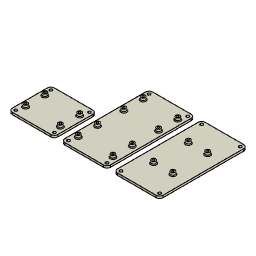
Lower Bay Tray - Parametric Mount Generator (Autodesk Fusion 360 design; units mm, degrees)
Autodesk Fusion 360 part; units mm, degrees
sketch "Base Sketch" plane through (0, 0, 0) normal (0, 0, 1) x (1, 0, 0)
  line L0 (-65, 70) -> (-10, 70) construction
  line L1 (-10, 70) -> (-10, 20) construction
  line L2 (-10, 20) -> (-65, 20) construction
  line L3 (-65, 20) -> (-65, 70) construction
  line L4 (-70, 20) -> (-70, 70)
  arc A0 (-65, 75) -> (-70, 70) centre (-65, 70) ccw
  arc A1 (-5, 70) -> (-10, 75) centre (-10, 70) ccw
  line L5 (-5, 70) -> (-5, 20)
  line L6 (-65, 75) -> (-10, 75)
  arc A2 (-70, 20) -> (-65, 15) centre (-65, 20) ccw
  line L7 (-10, 15) -> (-65, 15)
  arc A3 (-10, 15) -> (-5, 20) centre (-10, 20) ccw
  line L8 (-66.8, 70.25) -> (-66.8, 69.75)
  arc A4 (-66.8, 69.75) -> (-63.2, 69.75) centre (-65, 69.75) ccw
  line L9 (-63.2, 69.75) -> (-63.2, 70.25)
  arc A5 (-63.2, 70.25) -> (-66.8, 70.25) centre (-65, 70.25) ccw
  line L10 (-65, 70.25) -> (-65, 69.75) construction
  line L11 (-37.5, 75) -> (-37.5, 15) construction
  line L12 (-70, 45) -> (-5, 45) construction
  arc A6 (-66.8, 19.75) -> (-63.2, 19.75) centre (-65, 19.75) ccw
  line L13 (-66.8, 19.75) -> (-66.8, 20.25)
  arc A7 (-63.2, 20.25) -> (-66.8, 20.25) centre (-65, 20.25) ccw
  line L14 (-63.2, 20.25) -> (-63.2, 19.75)
  arc A8 (-8.2, 70.25) -> (-11.8, 70.25) centre (-10, 70.25) ccw
  line L15 (-8.2, 70.25) -> (-8.2, 69.75)
  arc A9 (-11.8, 69.75) -> (-8.2, 69.75) centre (-10, 69.75) ccw
  line L16 (-11.8, 69.75) -> (-11.8, 70.25)
  line L17 (-11.8, 20.25) -> (-11.8, 19.75)
  arc A10 (-8.2, 20.25) -> (-11.8, 20.25) centre (-10, 20.25) ccw
  line L18 (-8.2, 19.75) -> (-8.2, 20.25)
  arc A11 (-11.8, 19.75) -> (-8.2, 19.75) centre (-10, 19.75) ccw
  line L19 (70, 140) -> (70, 15) construction
  line L20 (70, 15) -> (5, 15) construction
  line L21 (5, 140) -> (70, 140) construction
  line L22 (5, 15) -> (5, 140) construction
  line L23 (10, 135) -> (65, 135) construction
  line L24 (65, 135) -> (65, 20) construction
  line L25 (65, 20) -> (10, 20) construction
  line L26 (10, 20) -> (10, 135) construction
  line L27 (65, 15) -> (10, 15)
  line L28 (5, 20) -> (5, 135)
  line L29 (10, 140) -> (65, 140)
  line L30 (70, 135) -> (70, 20)
  arc A12 (10, 140) -> (5, 135) centre (10, 135) ccw
  arc A13 (70, 135) -> (65, 140) centre (65, 135) ccw
  arc A14 (5, 20) -> (10, 15) centre (10, 20) ccw
  arc A15 (65, 15) -> (70, 20) centre (65, 20) ccw
  line L31 (8.1, 135.25) -> (8.1, 134.75)
  arc A16 (8.1, 134.75) -> (11.9, 134.75) centre (10, 134.75) ccw
  line L32 (11.9, 134.75) -> (11.9, 135.25)
  arc A17 (11.9, 135.25) -> (8.1, 135.25) centre (10, 135.25) ccw
  line L33 (10, 135.25) -> (10, 134.75) construction
  line L34 (37.5, 140) -> (37.5, 15) construction
  line L35 (5, 77.5) -> (70, 77.5) construction
  arc A18 (63.1, 134.75) -> (66.9, 134.75) centre (65, 134.75) ccw
  line L36 (63.1, 134.75) -> (63.1, 135.25)
  arc A19 (66.9, 135.25) -> (63.1, 135.25) centre (65, 135.25) ccw
  line L37 (66.9, 135.25) -> (66.9, 134.75)
  line L38 (66.9, 19.75) -> (66.9, 20.25)
  arc A20 (63.1, 19.75) -> (66.9, 19.75) centre (65, 19.75) ccw
  line L39 (63.1, 20.25) -> (63.1, 19.75)
  arc A21 (66.9, 20.25) -> (63.1, 20.25) centre (65, 20.25) ccw
  arc A22 (8.1, 19.75) -> (11.9, 19.75) centre (10, 19.75) ccw
  line L40 (8.1, 19.75) -> (8.1, 20.25)
  line L41 (11.9, 20.25) -> (11.9, 19.75)
  arc A23 (11.9, 20.25) -> (8.1, 20.25) centre (10, 20.25) ccw
  point P0 (-65, 70)
  point P1 (10, 135)
  point P2 (65, 135)
  point P3 (10, 20)
  point P4 (65, 20)
  point P5 (10, 135)
  dimension "d1" = 3.6
  dimension "d5" = 3.8
  constraint tangent L8 A4
  constraint tangent A4 L9
  constraint parallel L8 L9
  constraint tangent L9 A5
  constraint tangent L8 A5
  constraint vertical L10
  constraint coincident P0 L0.start
  constraint midpoint L10 P0
  constraint midpoint L6 L11.start
  constraint midpoint L7 L11.end
  constraint midpoint L4 L12.start
  constraint midpoint L5 L12.end
  constraint symmetric L8.start L12 A6.start
  constraint symmetric L8.end L12 L13.end
  constraint symmetric A4.end L12 A7.start
  constraint symmetric L9.end L12 A6.end
  constraint symmetric A4 L12 A7
  constraint symmetric A5 L12 A6
  constraint symmetric L8.start L11 A8.start
  constraint symmetric L8.end L11 L15.end
  constraint symmetric A4.end L11 A9.start
  constraint symmetric L9.end L11 A8.end
  constraint symmetric A4 L11 A9
  constraint symmetric A5 L11 A8
  constraint symmetric L11 A6.end L17.end
  constraint symmetric L11 A6.start L18.start
  constraint symmetric L11 A6 A11
  constraint symmetric L11 L13.end A10.start
  constraint symmetric L11 A7.start L17.start
  constraint symmetric L11 A7 A10
  constraint horizontal L23
  constraint vertical L24
  constraint horizontal L25
  constraint vertical L26
  constraint coincident P4 L24.end
  constraint coincident P5 P1
  constraint coincident L21 L29.start
  constraint parallel L25 L27
  constraint parallel L26 L28
  constraint parallel L23 L29
  constraint parallel L24 L30
  constraint coincident L21 L29.end
  constraint coincident P2 L23.end
  constraint coincident L22 L28.start
  constraint coincident P3 L25.end
  constraint tangent L31 A16
  constraint tangent A16 L32
  constraint parallel L31 L32
  constraint tangent L32 A17
  constraint tangent L31 A17
  constraint vertical L33
  constraint midpoint L33 P5
  constraint midpoint L21 L34.start
  constraint midpoint L20 L34.end
  constraint midpoint L28 L35.start
  constraint midpoint L19 L35.end
  constraint symmetric L31.start L34 A19.start
  constraint symmetric L31.end L34 A18.end
  constraint symmetric A16.end L34 A18.start
  constraint symmetric L32.end L34 L36.end
  constraint symmetric A16 L34 A18
  constraint symmetric A17 L34 A19
  constraint symmetric L31.start L35 A22.start
  constraint symmetric L31.end L35 L40.end
  constraint symmetric A16.end L35 L41.start
  constraint symmetric L32.end L35 A22.end
  constraint symmetric A16 L35 A23
  constraint symmetric A17 L35 A22
  constraint symmetric L35 A18.end L38.end
  constraint symmetric L35 A18.start L39.start
  constraint symmetric L35 A18 A21
  constraint symmetric L35 L36.end A20.start
  constraint symmetric L35 A19.start L38.start
  constraint symmetric L35 A19 A20
  measures "d1" diameter of A4
  measures "d5" diameter of A16
extrude "Extrude1" add sketch "Base Sketch" along normal blind 3 contours L4 A0 A1 L5 L6 A2 L7 A3 makes body 1 in component "Single Template"
extrude "Extrude1'" add sketch "Base Sketch" along normal blind 3 separate body contours L27 L28 L29 L30 A12 A13 A14 A15 makes body 2 in component "Large Dual Template"
ref_plane "WorkPlane1" through (0, 0, 3) normal (0, 0, 1) x (1, 0, 0)
sketch "Mounting Hole Generator" plane through (0, 0, 3) normal (0, 0, 1) x (1, 0, 0)
  arc A0 (-66.8, 19.75) -> (-63.2, 19.75) centre (-65, 19.75) ccw
  line L0 (-66.8, 19.75) -> (-66.8, 20.25)
  arc A1 (-63.2, 20.25) -> (-66.8, 20.25) centre (-65, 20.25) ccw
  line L1 (-63.2, 20.25) -> (-63.2, 19.75)
  arc A2 (-8.2, 70.25) -> (-11.8, 70.25) centre (-10, 70.25) ccw
  line L2 (-8.2, 70.25) -> (-8.2, 69.75)
  arc A3 (-11.8, 69.75) -> (-8.2, 69.75) centre (-10, 69.75) ccw
  line L3 (-11.8, 69.75) -> (-11.8, 70.25)
  arc A4 (-63.2, 70.25) -> (-66.8, 70.25) centre (-65, 70.25) ccw
  line L4 (-63.2, 70.25) -> (-63.2, 69.75)
  arc A5 (-66.8, 69.75) -> (-63.2, 69.75) centre (-65, 69.75) ccw
  line L5 (-66.8, 69.75) -> (-66.8, 70.25)
  arc A6 (-11.8, 19.75) -> (-8.2, 19.75) centre (-10, 19.75) ccw
  line L6 (-11.8, 19.75) -> (-11.8, 20.25)
  arc A7 (-8.2, 20.25) -> (-11.8, 20.25) centre (-10, 20.25) ccw
  line L7 (-8.2, 20.25) -> (-8.2, 19.75)
  arc A8 (-70, 20) -> (-65, 15) centre (-65, 20) ccw
  line L8 (-65, 15) -> (-10, 15)
  arc A9 (-10, 15) -> (-5, 20) centre (-10, 20) ccw
  line L9 (-5, 20) -> (-5, 70)
  arc A10 (-5, 70) -> (-10, 75) centre (-10, 70) ccw
  line L10 (-10, 75) -> (-65, 75)
  arc A11 (-65, 75) -> (-70, 70) centre (-65, 70) ccw
  line L11 (-70, 70) -> (-70, 20)
  arc A12 (66.9, 20.25) -> (63.1, 20.25) centre (65, 20.25) ccw
  line L12 (66.9, 20.25) -> (66.9, 19.75)
  arc A13 (63.1, 19.75) -> (66.9, 19.75) centre (65, 19.75) ccw
  line L13 (63.1, 19.75) -> (63.1, 20.25)
  arc A14 (11.9, 135.25) -> (8.1, 135.25) centre (10, 135.25) ccw
  line L14 (11.9, 135.25) -> (11.9, 134.75)
  arc A15 (8.1, 134.75) -> (11.9, 134.75) centre (10, 134.75) ccw
  line L15 (8.1, 134.75) -> (8.1, 135.25)
  arc A16 (8.1, 19.75) -> (11.9, 19.75) centre (10, 19.75) ccw
  line L16 (8.1, 19.75) -> (8.1, 20.25)
  arc A17 (11.9, 20.25) -> (8.1, 20.25) centre (10, 20.25) ccw
  line L17 (11.9, 20.25) -> (11.9, 19.75)
  arc A18 (63.1, 134.75) -> (66.9, 134.75) centre (65, 134.75) ccw
  line L18 (63.1, 134.75) -> (63.1, 135.25)
  arc A19 (66.9, 135.25) -> (63.1, 135.25) centre (65, 135.25) ccw
  line L19 (66.9, 135.25) -> (66.9, 134.75)
  arc A20 (5, 20) -> (10, 15) centre (10, 20) ccw
  line L20 (10, 15) -> (65, 15)
  arc A21 (65, 15) -> (70, 20) centre (65, 20) ccw
  line L21 (70, 20) -> (70, 135)
  arc A22 (70, 135) -> (65, 140) centre (65, 135) ccw
  line L22 (65, 140) -> (10, 140)
  arc A23 (10, 140) -> (5, 135) centre (10, 135) ccw
  line L23 (5, 135) -> (5, 20)
  line L24 (-37.5, 75) -> (-37.5, 15) construction
  line L25 (-70, 45) -> (-5, 45) construction
  line L26 (-12.75, 31.25) -> (-62.25, 31.25) construction
  line L27 (-62.25, 31.25) -> (-62.25, 58.75) construction
  line L28 (-62.25, 58.75) -> (-12.75, 58.75) construction
  line L29 (-12.75, 58.75) -> (-12.75, 31.25) construction
  line L30 (-12.75, 31.25) -> (-62.25, 58.75) construction
  line L31 (-62.25, 31.25) -> (-12.75, 58.75) construction
  circle A24 centre (-62.25, 58.75) radius 1.4
  circle A25 centre (-62.25, 58.75) radius 3
  circle A26 centre (-12.75, 58.75) radius 1.4
  circle A27 centre (-12.75, 58.75) radius 3
  circle A28 centre (-12.75, 31.25) radius 3
  circle A29 centre (-12.75, 31.25) radius 1.4
  circle A30 centre (-62.25, 31.25) radius 3
  circle A31 centre (-62.25, 31.25) radius 1.4
  line L32 (0, 0) -> (0, 20) construction
  line L33 (5, 77.5) -> (70, 77.5) construction
  circle A32 centre (62.25, 58.75) radius 3
  circle A33 centre (62.25, 58.75) radius 1.4
  circle A34 centre (12.75, 58.75) radius 1.4
  circle A35 centre (12.75, 58.75) radius 3
  circle A36 centre (12.75, 31.25) radius 3
  circle A37 centre (12.75, 31.25) radius 1.4
  circle A38 centre (62.25, 31.25) radius 3
  circle A39 centre (62.25, 31.25) radius 1.4
  circle A40 centre (62.25, 96.25) radius 1.4
  circle A41 centre (62.25, 96.25) radius 3
  circle A42 centre (62.25, 123.75) radius 1.4
  circle A43 centre (12.75, 123.75) radius 1.4
  circle A44 centre (12.75, 96.25) radius 1.4
  circle A45 centre (62.25, 123.75) radius 3
  circle A46 centre (12.75, 96.25) radius 3
  circle A47 centre (12.75, 123.75) radius 3
  point P0 (-37.5, 45)
  dimension "d14" = 49.5
  dimension "d15" = 27.5
  dimension "d16" = 2.8
  dimension "d17" = 1.6
  dimension "d18" = 2.8
  dimension "d19" = 1.6
  constraint midpoint L10 L24.start
  constraint midpoint L8 L24.end
  constraint midpoint L11 L25.start
  constraint perpendicular L11 L25
  constraint horizontal L26
  constraint perpendicular L26 L27
  constraint parallel L26 L28
  constraint parallel L27 L29
  constraint coincident L30 P0
  constraint coincident L31 P0
  constraint midpoint L25 P0
  constraint coincident L27.end L28.start
  constraint coincident L28.end L29.start
  constraint symmetric L25 A24 A31
  constraint symmetric L25 A25 A30
  constraint symmetric L25 A26 A29
  constraint symmetric L25 A27 A28
  constraint coincident L32.start origin
  constraint parallel L23 L32
  constraint midpoint L23 L33.start
  constraint midpoint L21 L33.end
  constraint symmetric A24 L32 A33
  constraint symmetric A25 L32 A32
  constraint symmetric A26 L32 A34
  constraint symmetric A27 L32 A35
  constraint symmetric A28 L32 A36
  constraint symmetric A29 L32 A37
  constraint symmetric A30 L32 A38
  constraint symmetric A31 L32 A39
  constraint symmetric L33 A32 A41
  constraint symmetric L33 A33 A40
  constraint symmetric L33 A34 A44
  constraint symmetric L33 A35 A46
  constraint symmetric L33 A36 A47
  constraint symmetric L33 A37 A43
  constraint symmetric L33 A38 A45
  constraint symmetric L33 A39 A42
  measures "d14" distance of L27.end L28.end
  measures "d15" distance of L26.end L27.end
  measures "d16" diameter of A24
  measures "d18" diameter of A26
copy_body "CopyPasteBodies1" bodies 2 makes body 3
move_body "Move1" bodies 3 to x (1, 0, 0) y (0, 1, 0) z (0, 0, 1) at (74.9, 0, 0)
copy_body "Body->Comp1" bodies 3 removing the originals makes body 4 in component "Large Single Template"
sketch "Sketch3" plane through (0, 0, 3) normal (0, 0, 1) x (-1, 0, 0)
  arc A0 (-141.8, -20.25) -> (-138, -20.25) centre (-139.9, -20.25) ccw
  line L0 (-141.8, -20.25) -> (-141.8, -19.75)
  arc A1 (-138, -19.75) -> (-141.8, -19.75) centre (-139.9, -19.75) ccw
  line L1 (-138, -19.75) -> (-138, -20.25)
  arc A2 (-86.8, -135.25) -> (-83, -135.25) centre (-84.9, -135.25) ccw
  line L2 (-86.8, -135.25) -> (-86.8, -134.75)
  arc A3 (-83, -134.75) -> (-86.8, -134.75) centre (-84.9, -134.75) ccw
  line L3 (-83, -134.75) -> (-83, -135.25)
  arc A4 (-83, -19.75) -> (-86.8, -19.75) centre (-84.9, -19.75) ccw
  line L4 (-83, -19.75) -> (-83, -20.25)
  arc A5 (-86.8, -20.25) -> (-83, -20.25) centre (-84.9, -20.25) ccw
  line L5 (-86.8, -20.25) -> (-86.8, -19.75)
  arc A6 (-138, -134.75) -> (-141.8, -134.75) centre (-139.9, -134.75) ccw
  line L6 (-138, -134.75) -> (-138, -135.25)
  arc A7 (-141.8, -135.25) -> (-138, -135.25) centre (-139.9, -135.25) ccw
  line L7 (-141.8, -135.25) -> (-141.8, -134.75)
  arc A8 (-79.9, -20) -> (-84.9, -15) centre (-84.9, -20) ccw
  line L8 (-84.9, -15) -> (-139.9, -15)
  arc A9 (-139.9, -15) -> (-144.9, -20) centre (-139.9, -20) ccw
  line L9 (-144.9, -20) -> (-144.9, -135)
  arc A10 (-144.9, -135) -> (-139.9, -140) centre (-139.9, -135) ccw
  line L10 (-139.9, -140) -> (-84.9, -140)
  arc A11 (-84.9, -140) -> (-79.9, -135) centre (-84.9, -135) ccw
  line L11 (-79.9, -135) -> (-79.9, -20)
  line L12 (-79.9, -77.5) -> (-144.9, -77.5) construction
  line L13 (-126.15, -52.75) -> (-98.65, -52.75) construction
  line L14 (-98.65, -52.75) -> (-98.65, -102.25) construction
  line L15 (-98.65, -102.25) -> (-126.15, -102.25) construction
  line L16 (-126.15, -102.25) -> (-126.15, -52.75) construction
  line L17 (-126.15, -52.75) -> (-98.65, -102.25) construction
  line L18 (-98.65, -52.75) -> (-126.15, -102.25) construction
  circle A12 centre (-98.65, -102.25) radius 1.4
  circle A13 centre (-98.65, -102.25) radius 3
  circle A14 centre (-126.15, -102.25) radius 1.4
  circle A15 centre (-126.15, -102.25) radius 3
  circle A16 centre (-126.15, -52.75) radius 1.4
  circle A17 centre (-126.15, -52.75) radius 3
  circle A18 centre (-98.65, -52.75) radius 1.4
  circle A19 centre (-98.65, -52.75) radius 3
  point P0 (-112.4, -77.5)
  dimension "d28" = 27.5
  dimension "d29" = 49.5
  dimension "d30" = 2.8
  dimension "d31" = 1.6
  dimension "d32" = 2.8
  dimension "d33" = 1.6
  dimension "d34" = 1.6
  dimension "d35" = 2.8
  dimension "d36" = 2.8
  dimension "d37" = 1.6
  constraint midpoint L11 L12.start
  constraint midpoint L9 L12.end
  constraint horizontal L13
  constraint perpendicular L13 L14
  constraint parallel L13 L15
  constraint parallel L14 L16
  constraint coincident L17 P0
  constraint coincident L18 P0
  constraint midpoint L12 P0
  constraint coincident L14.end L15.start
  constraint coincident L15.end L16.start
  constraint coincident L13.start L16.end
  constraint coincident L13.end L14.start
  measures "d28" distance of L14.end L15.end
  measures "d29" distance of L13.end L14.end
  measures "d30" diameter of A12
  measures "d32" diameter of A14
  measures "d35" diameter of A16
  measures "d36" diameter of A18
extrude "Extrude1''" add sketch "Sketch3" along normal blind 4 contours A13 | A15 | A17 | A19 bodies 4 in component "Large Single Template"
fillet "Fillet1" radius 1 4 edges at (101.447, 51.6652, 3) (101.447, 101.1652, 3) (128.947, 51.6652, 3) (128.947, 101.1652, 3) on bodies 4 in component "Large Single Template"
extrude "Extrude2" add sketch "Mounting Hole Generator" along normal blind 4 contours A25 | A27 | A28 | A30 bodies 1 in component "Single Template"
fillet "Fillet1'" radius 1 4 edges at (-65.047, 32.3348, 3) (-65.047, 59.8348, 3) (-15.547, 59.8348, 3) (-15.547, 32.3348, 3) on bodies 1 in component "Single Template"
extrude "Extrude2'" add sketch "Mounting Hole Generator" along normal blind 4 contours A32 | A35 | A36 | A38 | A41 | A45 | A46 | A47 bodies 2 in component "Large Dual Template"
fillet "Fillet1''" radius 1 8 edges at (9.953, 59.8348, 3) (59.453, 32.3348, 3) (9.953, 32.3348, 3) (59.453, 59.8348, 3) (9.953, 97.3348, 3) (9.953, 124.8348, 3) (59.453, 97.3348, 3) (59.453, 124.8348, 3) on bodies 2 in component "Large Dual Template"
component "Single Template" placed x (1, 0, 0) y (0, 1, 0) z (0, 0, 1) at (0, 0, 0)
component "Large Dual Template" placed x (1, 0, 0) y (0, 1, 0) z (0, 0, 1) at (0, 0, 0)
component "Large Single Template" placed x (1, 0, 0) y (0, 1, 0) z (0, 0, 1) at (0, 0, 0)
equation "short_len = 27.5 mm" comment "Shorter side of the mounting hole rect"
equation "long_len = 49.5 mm" comment "Larger side of the mounting hole rect"
equation "hole_dia = 2.8 mm" comment "Mounting hole diameter"
equation "d14 = long_len"
equation "d15 = short_len"
equation "d16 = hole_dia"
equation "d18 = hole_dia"
equation "d28 = short_len"
equation "d29 = long_len"
equation "d30 = d32"
equation "d35 = d32"
equation "d36 = d35"
